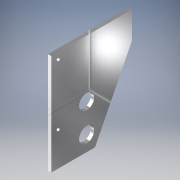
# Autodesk Inventor part: 15102898-16-P-0302
Saved by Autodesk Inventor 2017 (Build 210142000, 142)
## iProperties
Created: 2016-10-02
Part Number: 15102898-16-P-0302
Material: Aluminum 6061
Document SubType Name: Sheet Metal
Designer: gus
Density: 2.7 g/cm^3
Appearance: Aluminum - Flat
Sheet Metal Rule: Default
Author: gus
Autodesk Inventor part; units mm, degrees
ref_plane "YZ Plane" through (0, 0, 0) normal (1, 0, 0) x (0, 1, 0)
ref_plane "XZ Plane" through (0, 0, 0) normal (0, 1, 0) x (-1, 0, 0)
ref_plane "XY Plane" through (0, 0, 0) normal (0, 0, 1) x (1, 0, 0)
sketch "Sketch1" plane through (0, 0, 0) normal (1, 0, 0) x (0, 1, 0)
  line L0 (0, 0) -> (63.5, 0)
  line L1 (63.5, 0) -> (63.5, -127)
  line L2 (63.5, -127) -> (12.7, -127)
  circle A0 centre (-31.75, -53.975) radius 14.2875
  line L3 (63.5, -25.4) -> (-43.502, -25.4) construction
  circle A1 centre (50.8, -12.7) radius 3.175
  circle A2 centre (-50.8, -12.7) radius 3.175
  line L4 (12.7, -127) -> (-114.3, -69.85)
  line L5 (-114.3, -69.85) -> (-114.3, 0)
  line L6 (-114.3, 0) -> (0, 0)
  circle A3 centre (-85.725, -53.975) radius 14.2875
  dimension "d1" = 28.575
  dimension "d2" = 63.5
  dimension "d6" = 25.4
  dimension "d7" = 6.35
  dimension "d8" = 6.35
  dimension "d9" = 12.7
  dimension "d10" = 12.7
  dimension "d12" = 12.7
  dimension "d17" = 50.8
  dimension "d18" = 114.3
  dimension "d19" = 63.5
  dimension "d20" = 53.975
  dimension "d21" = 28.575
  dimension "d24" = 53.975
  dimension "d25" = 69.85
  dimension "d26" = 53.975
  dimension "d27" = 127
  dimension "d28" = 107.002
  constraints: 14 end point, 4 centre point, 2 perpendicular, 1 collinear, 1 equal radius, 1 horizontal, 1 parallel, 1 point on line
  measures "d1" diameter of A0
  measures "d2" distance of L0.start L0.end
  measures "d6" distance between parallel lines of L0 L3
  measures "d7" diameter of A1
  measures "d8" diameter of A2
  measures "d9" distance from line of L3 A2.centre
  measures "d10" distance from line of L3 A1.centre
  measures "d12" distance from line of L1 A1.centre
  measures "d17" distance of L1.end L2.end
  measures "d18" distance from line of L0.start L5
  measures "d19" distance from line of L5 A2.centre
  measures "d20" distance from line of L6 A3.centre
  measures "d21" distance from line of L5 A3.centre
  measures "d24" distance from line of L0 A0.centre
  measures "d25" distance of L4.end L5.end
  measures "d26" distance of A3.centre A0.centre
  measures "d27" distance of L0.end L1.end
  measures "d28" distance of L3.start L3.end
extrude "Extrusion1" add sketch "Sketch1" along normal blind 6.35 contours L0 L1 L2 L4 L5 L6 | A3
extrude "Extrusion2" cut sketch "Sketch1" along normal blind 25.4 contours A3
equation "\"BendRadius\" = Thickness"
equation "\"BendReliefWidth\" = Thickness"
equation "\"BendReliefDepth\" = 0.5 * Thickness"
equation "\"CornerReliefSize\" = 4 * Thickness"
equation "\"MinimumRemnant\" = 2 * Thickness"
equation "\"TransitionRadius\" = BendRadius"
equation "\"JacobiRadiusSize\" = Thickness"
equation "\"GapSize\" = Thickness"
equation "\"Thickness\" = 3.048"
body "Solid1"
